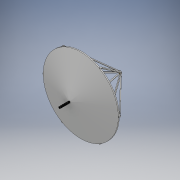
# Autodesk Inventor part: Dish
Saved by Autodesk Inventor 2018.3 (Build 223284000, 284)
## iProperties
Created: 2020-03-31
Part Number: Dish
Material: Generic
Document SubType Name: Modeling
Designer: ToreDenStore
Density: 1 g/cm^3
Appearance: Default
Author: ToreDenStore
Autodesk Inventor part; units mm, degrees
ref_plane "YZ Plane" through (0, 0, 0) normal (1, 0, 0) x (0, 1, 0)
ref_plane "XZ Plane" through (0, 0, 0) normal (0, 1, 0) x (-1, 0, 0)
ref_plane "XY Plane" through (0, 0, 0) normal (0, 0, 1) x (1, 0, 0)
sketch "Sketch1" plane through (0, 0, 0) normal (0, 0, 1) x (1, 0, 0)
  line L0 (0, 0) -> (-20, 0)
  line L1 (0, 0) -> (0, 917.6078) construction
  line L2 (0, 0) -> (0, -100)
  line L3 (0, 0) -> (100, 0) construction
  line L4 (0, -100) -> (-20, -100)
  line L5 (-20, -100) -> (-20, 0)
  arc A0 (-765.3669, 152.2409) -> (0, 0) centre (0, 2000) ccw
  line L6 (0, 2000) -> (-765.3669, 152.2409) construction
  line L7 (0, 2000) -> (0, 0) construction
  line L8 (0, -520) -> (0, 2420) projected
  line L9 (-765.3669, 152.2409) -> (-765.3669, 1234.6331) construction
  line L10 (-765.3669, 152.2409) -> (0, 917.6078) construction
  line L11 (0, 917.6078) -> (-92.388, 955.8761) construction
  line L12 (0, 917.6078) -> (92.388, 879.3395) construction
  arc A1 (0, 917.6078) -> (-20, 921.586) centre (-20, 869.3235) ccw
  line L13 (0, 917.6078) -> (-20, 869.3235) construction
  line L14 (-20, 921.586) -> (-20, 869.3235) construction
  line L15 (-20, 921.586) -> (-20, 941.586)
  line L16 (-20, 941.586) -> (0, 941.586)
  line L17 (0, 917.6078) -> (0, 941.586)
  line L18 (-765.3669, 152.2409) -> (-765.3669, 132.2409)
  line L19 (-765.3669, 132.2409) -> (-20, -100)
  dimension "d0" = 20
  dimension "d2" = 100
  dimension "d3" = 90
  dimension "d5" = 22.5
  dimension "d6" = 2000
  dimension "d7" = 22.5
  dimension "d8" = 22.5
  dimension "d9" = 1082.3922
  dimension "d11" = 45
  dimension "d12" = 917.6078
  dimension "d13" = 100
  dimension "d14" = 67.5
  dimension "d19" = 100
  dimension "d21" = 22.5
  dimension "d22" = 20
  dimension "d23" = 20
  dimension "d24" = 20
  constraints: 38 end point, 4 perpendicular, 4 point on circle, 4 vertical, 2 centre point, 2 collinear, 2 equal length, 2 horizontal, 2 point on line, 1 coincident, 1 parallel, 1 tangent
  measures "d0" distance of L0.start L0.end
  measures "d2" distance of L0.start L2.end
  measures "d3" angle of L2 L3
  measures "d5" angle of L6 L7
  measures "d6" distance of L6.start L0.start
  measures "d7" angle of L6 L9
  measures "d8" angle of L6 L10
  measures "d9" distance of L6.end L9.end
  measures "d11" angle of L1 L10
  measures "d12" distance of L0.start L1.end
  measures "d13" distance of L1.end L11.end
  measures "d14" angle of L11 L10
  measures "d19" distance of L1.end L12.end
  measures "d21" angle of L13 L14
  measures "d22" distance from line of L8 L14.start
  measures "d23" distance of L14.start L15.end
  measures "d24" distance of L6.end L18.end
revolve "Revolution1" add sketch "Sketch1" angle 360 about axis through (0, -10, 0) along (0, 1, 0) contours L0 L5 L19 L18 A0 | A1 L15 L16 L8
sketch "Sketch2" plane through (0, 0, 0) normal (0, 0, 1) x (1, 0, 0)
  line L0 (765.3669, 152.2409) -> (-765.3669, 152.2409) projected
  line L1 (20, 921.586) -> (-20, 921.586) projected
  line L2 (-765.3669, 152.2409) -> (-20, 921.586)
  line L3 (-20, 921.586) -> (-20, 941.586) projected
  line L4 (20, 941.586) -> (-20, 941.586) projected
  line L5 (-20, 921.586) -> (-20, 941.586)
  line L6 (-20, 941.586) -> (-765.3669, 172.2409)
  line L7 (-765.3669, 172.2409) -> (-765.3669, 152.2409)
  point P0 (0, 0)
  dimension "d26" = 20
  constraints: 8 end point, 1 parallel, 1 vertical
  measures "d26" distance of L6.end L0.end
extrude "Extrusion1" add sketch "Sketch2" along normal mid plane 20
sketch "Sketch3" plane through (-765.3669, 152.2409, 10) normal (-1, 0, 0) x (0, 0, 1)
  line L0 (0, 0) -> (-10, 0) projected
  line L1 (0, 20) -> (0, 0) projected
  line L2 (-20, 20) -> (0, 20) projected
  line L3 (-20, 0) -> (-20, 20) projected
  line L4 (-10, 0) -> (-20, 0) projected
  line L5 (-20, 20) -> (0, 20)
  line L6 (0, 20) -> (0, -20)
  line L7 (0, 0) -> (0, 769.3451) projected
  line L8 (0, -20) -> (-20, -20)
  line L9 (755.3669, -20) -> (-775.3669, -20) projected
  line L10 (-20, 20) -> (-20, 789.3451) projected
  line L11 (-20, 20) -> (-20, -20)
  point P0 (-10, -152.2409)
  dimension "d29" = 40
  constraints: 8 end point, 2 collinear, 1 perpendicular, 1 point on line
  measures "d29" distance of L1.start L6.end
extrude "Extrusion2" add sketch "Sketch3" along normal mid plane 20
sketch "Sketch4" plane through (-20, 921.586, 0) normal (1, 0, 0) x (0, 0, 1)
  line L0 (-10, 749.3451) -> (10, 749.3451) projected
  line L1 (10, -20) -> (10, 749.3451) construction
  line L2 (0, -20) -> (10, -20) projected
  line L3 (-10, -20) -> (0, -20) projected
  line L4 (-10, 749.3451) -> (-10, -20) construction
  line L5 (-10, 0) -> (-10, 759.0234) construction
  line L6 (-10, -20) -> (-10, 0)
  line L7 (-10, 0) -> (10, 0)
  line L8 (10, -20) -> (10, 749.3451) construction
  line L9 (10, -20) -> (-10, -20)
  line L10 (10, -20) -> (10, 0)
  point P0 (0, 921.586)
  constraints: 8 end point, 2 vertical, 1 collinear, 1 perpendicular, 1 point on line
extrude "Extrusion3" add sketch "Sketch4" along normal mid plane 20
pattern_circular "Circular Pattern1" count 6 over 360 about axis through (0, -50, 0) along (0, 1, 0) of "Extrusion1", "Extrusion2", "Extrusion3"
sketch "Sketch5" plane through (0, 0, 0) normal (0, 1, 0) x (-1, 0, 0)
  circle A0 centre (0, 0) radius 20 projected
extrude "Extrusion4" cut sketch "Sketch5" along normal blind 20
sketch "Sketch6" plane through (0, 0, 0) normal (0, 1, 0) x (-1, 0, 0)
  circle A0 centre (0, 0) radius 20 projected
extrude "Extrusion5" add sketch "Sketch6" against normal blind 300 separate body
equation "\"d8\" = d7"
body "Solid1"
body "Solid2"
